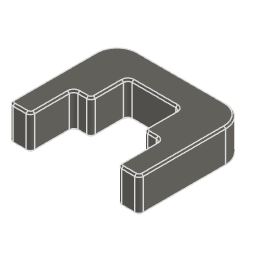
mgn12_rail_guide_x2 (Autodesk Fusion 360 design; units mm, degrees)
Autodesk Fusion 360 part; units mm, degrees
sketch "Sketch1" plane through (0, 0, 0) normal (0, 0, 1) x (1, 0, 0)
  line L0 (-6.05, -8.5) -> (-6.05, 0)
  line L1 (-6.05, 0) -> (6.05, 0)
  line L2 (6.05, 0) -> (6.05, -8.5)
  line L3 (6.05, -8.5) -> (10.05, -8.5)
  line L4 (10.05, -8.5) -> (10.05, -18.5)
  line L5 (-6.05, -8.5) -> (-10.05, -8.5)
  line L6 (-10.05, -8.5) -> (-10.05, -18.5)
  line L7 (10.05, -18.5) -> (15.05, -18.5)
  line L8 (15.05, -18.5) -> (15.05, 6.5)
  line L9 (15.05, 6.5) -> (-15.05, 6.5)
  line L10 (-15.05, 6.5) -> (-15.05, -18.5)
  line L11 (-15.05, -18.5) -> (-10.05, -18.5)
  arc A0 (-10.05, 6.5) -> (-15.05, 1.5) centre (-10.05, 1.5) ccw
  arc A1 (15.05, 1.5) -> (10.05, 6.5) centre (10.05, 1.5) ccw
  line L12 (-10.05, -18.5) -> (10.05, -18.5) construction
  point P0 (0, -18.5)
  dimension "d1" = 12.1
  dimension "d2" = 8.5
  dimension "d3" = 20.1
  dimension "d4" = 10
  dimension "d5" = 5
  dimension "d6" = 25
  dimension "d7" = 5
  dimension "d8" = 5
  constraint vertical L0
  constraint vertical L2
  constraint horizontal L1
  constraint coincident L0.start L5.start
  constraint horizontal L5
  constraint vertical L6
  constraint vertical L4
  constraint horizontal L3
  constraint horizontal L9
  constraint vertical L10
  constraint horizontal L11
  constraint horizontal L7
  constraint vertical L8
  constraint equal L0 L2
  constraint equal L4 L6
  constraint equal L7 L11
  constraint midpoint origin L1
  constraint coincident L9 A0.start
  constraint coincident L10 A0.end
  constraint tangent L9 A0
  constraint tangent L10 A0
  constraint coincident L9 A1.end
  constraint coincident L8 A1.start
  constraint tangent L9 A1
  constraint tangent L8 A1
  constraint midpoint L12 P0
  constraint vertical origin P0
  measures "d1" distance of L0 L2
  measures "d2" distance of L1.end L2.end
  measures "d3" distance of L4 L6
  measures "d4" distance of L3.end L4.end
  measures "d5" distance of L6.end L10.end
  measures "d6" distance of L7.end L8.end
  measures "d7" radius of A0
  measures "d8" radius of A1
extrude "Extrude1" add sketch "Sketch1" along normal blind 8 contours L0 L1 L2 L3 L4 L5 L6 L7 L8 L9 L10 L11 A0 A1
fillet "Fillet1" radius 1 10 edges at (6.05, 0, 4) (-6.05, 0, 4) (-6.05, -8.5, 4) (-10.05, -8.5, 4) (-10.05, -18.5, 4) (-15.05, -18.5, 4) (6.05, -8.5, 4) (10.05, -8.5, 4) (10.05, -18.5, 4) (15.05, -18.5, 4)
chamfer "Chamfer1" distance 0.4 angle 45 48 edges at (12.55, -18.5, 0) (14.7571, -18.2071, 0) (15.05, -8, 0) (13.5855, 5.0355, 0) (0, 6.5, 0) (-13.5855, 5.0355, 0) (-15.05, -8, 0) (-14.7571, -18.2071, 0) (-12.55, -18.5, 0) (-10.3429, -18.2071, 0) (-10.05, -13.5, 0) (-9.7571, -8.7929, 0) (-8.05, -8.5, 0) (-6.3429, -8.2071, 0) (-6.05, -4.25, 0) (-5.7571, -0.2929, 0) (0, 0, 0) (5.7571, -0.2929, 0) (6.05, -4.25, 0) (6.3429, -8.2071, 0) (8.05, -8.5, 0) (9.7571, -8.7929, 0) (10.05, -13.5, 0) (10.3429, -18.2071, 0) (12.55, -18.5, 8) (14.7571, -18.2071, 8) (15.05, -8, 8) (13.5855, 5.0355, 8) (0, 6.5, 8) (-13.5855, 5.0355, 8) (-15.05, -8, 8) (-14.7571, -18.2071, 8) (-12.55, -18.5, 8) (-10.3429, -18.2071, 8) (-10.05, -13.5, 8) (-9.7571, -8.7929, 8) (-8.05, -8.5, 8) (-6.3429, -8.2071, 8) (-6.05, -4.25, 8) (-5.7571, -0.2929, 8) (0, 0, 8) (5.7571, -0.2929, 8) (6.05, -4.25, 8) (6.3429, -8.2071, 8) (8.05, -8.5, 8) (9.7571, -8.7929, 8) (10.05, -13.5, 8) (10.3429, -18.2071, 8)
